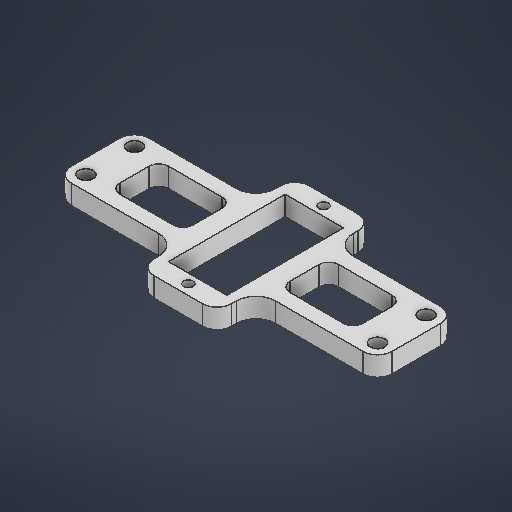
# Autodesk Inventor part: microservo_support1
Saved by Autodesk Inventor 2026.1 (Build 301233000, 233)
## iProperties
Created: 2025-10-17
Part Number: microservo_support1
Material: Generic
Document SubType Name: Modeling
Designer: emanuel
Density: 1 g/cm^3
Appearance: Default
Author: emanuel
Autodesk Inventor part; units mm, degrees
ref_plane "YZ Plane" through (0, 0, 0) normal (1, 0, 0) x (0, 1, 0)
ref_plane "XZ Plane" through (0, 0, 0) normal (0, 1, 0) x (-1, 0, 0)
ref_plane "XY Plane" through (0, 0, 0) normal (0, 0, 1) x (1, 0, 0)
sketch "Sketch1" plane through (0, 0, 0) normal (0, 1, 0) x (-1, 0, 0)
  line L0 (0, 0) -> (60, 0)
  line L1 (60, 0) -> (60, -10)
  line L2 (60, -10) -> (0, -10)
  line L3 (0, -10) -> (0, 0)
  circle A0 centre (60, 0) radius 1.5
  circle A1 centre (60, -10) radius 1.5
  circle A2 centre (0, 0) radius 1.5
  circle A3 centre (0, -10) radius 1.5
  line L4 (60, -10) -> (63, -10)
  line L5 (63, -10) -> (63, -13)
  line L6 (63, -13) -> (60, -13)
  line L7 (60, -13) -> (60, -10)
  line L8 (0, 0) -> (-3, 0)
  line L9 (-3, 0) -> (-3, 3)
  line L10 (-3, 3) -> (0, 3)
  line L11 (0, 3) -> (0, 0)
  line L12 (-3, 3) -> (63, 3)
  line L13 (63, 3) -> (63, -13)
  line L14 (63, -13) -> (-3, -13)
  line L15 (-3, -13) -> (-3, 3)
  line L16 (60, -5) -> (0, -5)
  line L17 (24, 7) -> (36, 7)
  line L18 (36, 7) -> (36, -17)
  line L19 (36, -17) -> (24, -17)
  line L20 (24, -17) -> (24, 7)
  line L21 (24, 7) -> (36, -17) construction
  line L22 (36, 7) -> (24, -17) construction
  line L23 (30, -5) -> (30, 6.25)
  line L24 (30, 6.25) -> (30, 8.9)
  circle A4 centre (30, 8.9) radius 1
  line L25 (30, -5) -> (30, -16.25)
  line L26 (30, -16.25) -> (30, -18.9)
  circle A5 centre (30, -18.9) radius 1
  line L27 (36, 7) -> (24, 7)
  line L28 (24, 7) -> (24, 11)
  line L29 (24, 11) -> (36, 11)
  line L30 (36, 11) -> (36, 7)
  line L31 (36, -17) -> (24, -17)
  line L32 (24, -17) -> (24, -21)
  line L33 (24, -21) -> (36, -21)
  line L34 (36, -21) -> (36, -17)
  line L35 (36, 11) -> (38, 11)
  line L36 (38, 11) -> (38, -21)
  line L37 (38, -21) -> (36, -21)
  line L38 (36, -21) -> (36, 11)
  line L39 (24, 11) -> (20.9428, 11)
  line L40 (24, 9) -> (24, 11)
  line L41 (24, 11) -> (22, 11)
  line L42 (22, 11) -> (22, -21)
  line L43 (22, -21) -> (24, -21)
  line L44 (24, -21) -> (24, 11)
  line L45 (60, -5) -> (55, -5)
  line L46 (55, -5) -> (40, -5)
  line L47 (40, -5) -> (40, 0)
  line L48 (40, 0) -> (55, 0)
  line L49 (55, 0) -> (55, -5)
  line L50 (55, 0) -> (40, 0)
  line L51 (40, 0) -> (40, -10)
  line L52 (40, -10) -> (55, -10)
  line L53 (55, -10) -> (55, 0)
  line L54 (0, -5) -> (5, -5)
  line L55 (5, -5) -> (20, -5)
  line L56 (20, -5) -> (20, 0)
  line L57 (20, 0) -> (5, 0)
  line L58 (5, 0) -> (5, -5)
  line L59 (20, 0) -> (5, 0)
  line L60 (5, 0) -> (5, -10)
  line L61 (5, -10) -> (20, -10)
  line L62 (20, -10) -> (20, 0)
  point P0 (24, -13)
  point P1 (24, 3)
  point P2 (38, 3)
  point P3 (38, -13)
  point P4 (22, -13)
  point P5 (22, 3)
  dimension "d0" = 60
  dimension "d1" = 10
  dimension "d2" = 3
  dimension "d3" = 3
  dimension "d4" = 3
  dimension "d5" = 3
  dimension "d6" = 3
  dimension "d7" = 3
  dimension "d8" = 3
  dimension "d9" = 3
  dimension "d12" = 12
  dimension "d13" = 24
  dimension "d14" = 11.25
  dimension "d15" = 2.65
  dimension "d16" = 2
  dimension "d17" = 11.25
  dimension "d18" = 2.65
  dimension "d19" = 2
  dimension "d20" = 4
  dimension "d21" = 4
  dimension "d22" = 2
  dimension "d24" = 2
  dimension "d28" = 5
  dimension "d29" = 15
  dimension "d30" = 5
  dimension "d31" = 5
  dimension "d32" = 15
  constraints: 126 end point, 27 parallel, 14 horizontal, 13 perpendicular, 11 point on line, 6 centre point, 6 coincident, 5 midpoint
  measures "d0" distance of L1.end L2.end
  measures "d1" distance of L0.end L1.end
  measures "d2" diameter of A0
  measures "d3" diameter of A1
  measures "d4" diameter of A2
  measures "d5" diameter of A3
  measures "d6" distance of L5.end L6.end
  measures "d7" distance of L4.end L5.end
  measures "d8" distance of L9.end L10.end
  measures "d9" distance of L8.end L9.end
  measures "d12" distance of L18.end L19.end
  measures "d13" distance of L17.end L18.end
  measures "d14" distance of L23.start L23.end
  measures "d15" distance of L23.end L24.end
  measures "d16" diameter of A4
  measures "d17" distance of L23.start L25.end
  measures "d18" distance of L25.end L26.end
  measures "d19" diameter of A5
  measures "d20" distance of L27.end L28.end
  measures "d21" distance of L32.end L31.end
  measures "d22" distance of L36.end L37.end
  measures "d24" distance of L43.end L42.end
  measures "d28" distance of L16.start L45.end
  measures "d29" distance of L47.end L48.end
  measures "d30" distance of L46.end L47.end
  measures "d31" distance of L16.end L54.end
  measures "d32" distance of L57.end L56.end
extrude "Extrusion1" add sketch "Sketch1" along normal blind 4 contours A2 L11 L12 L42 L0 | L0 L58 L16 L3 A2 | L3 A3 L2 L42 L14 L15 L8 A2 | L8 L9 L10 L11 A2 | L16 L60 L2 A3 L3 | L0 L42 L16 L56 | L42 L39 L28 L20 L12 | L12 L20 L0 L42 | L0 L20 L16 L42 | L16 L42 L2 L62 | L42 L2 L20 L14 | L14 L20 L32 L43 L42 | L16 L20 L2 L42 | L28 L29 L30 L17 | L19 L34 L33 L32 | L18 L30 L35 L36 L12 | L12 L36 L0 L18 | L0 L36 L16 L18 | L18 L2 L36 L14 | L14 L36 L37 L34 L18 | L12 L13 L4 A1 L1 A0 L0 L36 | L0 L47 L16 L36 | L16 L36 L2 L18 | L36 L2 A1 L7 L14 | L16 L51 L2 L36 | L7 A1 L4 L5 L6 | L0 A0 L1 L16 L49 | L16 L1 A1 L2 L53
fillet "Fillet1" radius 4 4 edges at (-22, 2, 3) (-22, 2, -13) (-38, 2, -13) (-38, 2, 3)
fillet "Fillet2" radius 3 4 edges at (-38, 2, 11) (-22, 2, 11) (-22, 2, -21) (-38, 2, -21)
fillet "Fillet3" radius 3 4 edges at (-63, 2, 3) (-63, 2, -13) (3, 2, -13) (3, 2, 3)
fillet "Fillet4" radius 2 8 edges at (-55, 2, -10) (-40, 2, -10) (-40, 2, 0) (-55, 2, 0) (-20, 2, -10) (-20, 2, 0) (-5, 2, 0) (-5, 2, -10)
body "Solid1"
